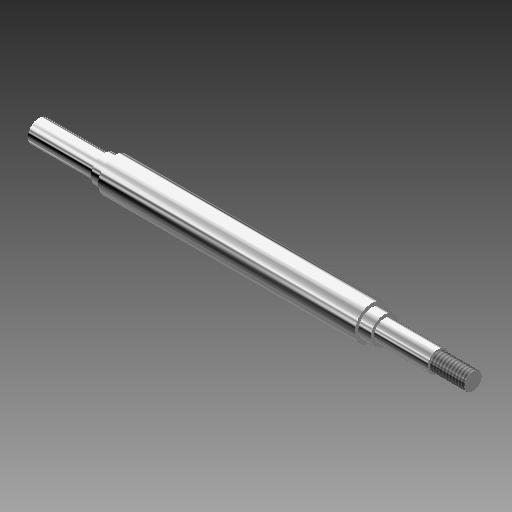
# Autodesk Inventor part: 401-05
Saved by Autodesk Inventor 2019 (Build 230136000, 136)
## iProperties
Company: Autodesk Inc.
Created: 2017-06-27
Part Number: 401-05
Material: Aluminum-6061
Document SubType Name: Modeling
Designer: Autodesk Inc.
Mass: 2.3605 g
Surface Area: 8.8293 cm^2
Volume: 0.874258 cm^3
Density: 2.7 g/cm^3
Appearance: Chrome - Polished
Author: Inventor
Autodesk Inventor part; units mm, degrees
ref_plane "YZ Plane" through (0, 0, 0) normal (1, 0, 0) x (0, 1, 0)
ref_plane "XZ Plane" through (0, 0, 0) normal (0, 1, 0) x (-1, 0, 0)
ref_plane "XY Plane" through (0, 0, 0) normal (0, 0, 1) x (1, 0, 0)
sketch "Sketch1" plane through (0, 0, 0) normal (0, 0, 1) x (1, 0, 0)
  line L0 (-18.4, 0) -> (18.4, 0)
  line L1 (18.4, 0) -> (18.4, 2.45)
  line L2 (18.4, 2.45) -> (-18.4, 2.45)
  line L3 (-18.4, 2.45) -> (-18.4, 0)
  line L4 (-18.4, 0) -> (-19.9, 0)
  line L5 (-19.9, 0) -> (-19.9, 1.95)
  line L6 (-19.9, 1.95) -> (-18.4, 1.95)
  line L7 (-18.4, 1.95) -> (-18.4, 0)
  line L8 (-19.9, 0) -> (-29.3, 0)
  line L9 (-29.3, 0) -> (-29.3, 1.6)
  line L10 (-29.3, 1.6) -> (-19.9, 1.6)
  line L11 (-19.9, 1.6) -> (-19.9, 0)
  line L12 (18.4, 0) -> (20.2, 0)
  line L13 (20.2, 0) -> (20.2, 1.95)
  line L14 (20.2, 1.95) -> (18.4, 1.95)
  line L15 (18.4, 1.95) -> (18.4, 0)
  line L16 (20.2, 0) -> (27.9, 0)
  line L17 (27.9, 0) -> (27.9, 1.5)
  line L18 (27.9, 1.5) -> (20.2, 1.5)
  line L19 (20.2, 1.5) -> (20.2, 0)
  line L20 (27.9, 0) -> (32.9, 0)
  line L21 (32.9, 0) -> (32.9, 1.25)
  line L22 (32.9, 1.25) -> (27.9, 1.25)
  line L23 (27.9, 1.25) -> (27.9, 0)
  point P0 (0, 0)
  point P1 (0, 0)
  dimension "d0" = 9.4
  dimension "d1" = 10.9
  dimension "d2" = 47.7
  dimension "d3" = 3.2
  dimension "d4" = 3.9
  dimension "d5" = 4.9
  dimension "d6" = 3
  dimension "d7" = 49.5
  dimension "d21" = 2.5
  dimension "d22" = 62.2
  dimension "d23" = 5
  constraints: 48 end point, 12 parallel, 6 horizontal, 6 perpendicular, 1 coincident, 1 collinear, 1 midpoint
  measures "d0" distance of L9.end L10.end
  measures "d1" distance between parallel lines of L3 L9
  measures "d2" distance between parallel lines of L1 L9
  measures "d3" diameter of L10 L8
  measures "d4" diameter of L6 L8
  measures "d5" diameter of L2 L8
  measures "d6" diameter of L18 L16
  measures "d7" distance between parallel lines of L19 L9
  measures "d21" diameter of L22 L20
  measures "d22" distance between parallel lines of L9 L21
  measures "d23" distance of L21.end L22.end
revolve "Revolution1" add sketch "Sketch1" angle 360 about axis through (-18.4, 0, 0) along (1, 0, 0)
thread "Thread1" size "M2.5x0.45" class "6g" standard "ANSI Metric M Profile" length 5
hole "Hole1" at (-29.3, 0, 0) direction (1, 0, 0) diameter 1.567 depth 6 tip angle 118 counterbore diameter 1.9 counterbore depth 2 thread size "M2x0.4" class "6H" standard "ANSI Metric M Profile"
body "Solid1"
